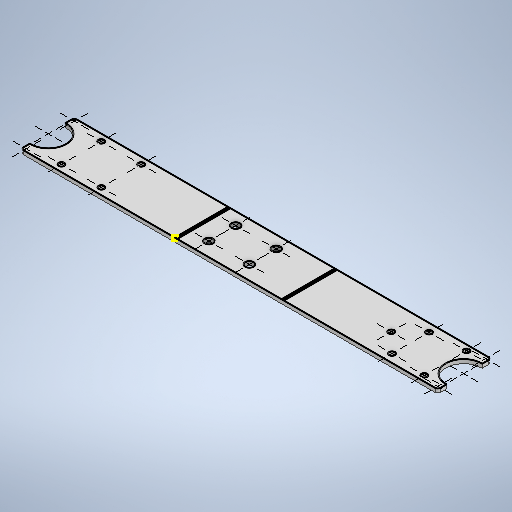
# Autodesk Inventor part: axis_21_top_frame
Saved by Autodesk Inventor 2026.1 (Build 301233000, 233)
## iProperties
Created: 2025-08-22
Part Number: axis_21_top_frame
Material: Generic
Document SubType Name: Modeling
Designer: LG
Density: 1 g/cm^3
Appearance: Default
Author: LG
Autodesk Inventor part; units mm, degrees
ref_plane "YZ Plane" through (0, 0, 0) normal (1, 0, 0) x (0, 1, 0)
ref_plane "XZ Plane" through (0, 0, 0) normal (0, 1, 0) x (-1, 0, 0)
ref_plane "XY Plane" through (0, 0, 0) normal (0, 0, 1) x (1, 0, 0)
sketch "Sketch1" plane through (0, 0, 0) normal (0, 1, 0) x (-1, 0, 0)
  line L0 (-40.8289, 0) -> (-40.8289, -20.14)
  line L1 (-0.4496, -20.14) -> (-0.4496, 0)
  circle A0 centre (45.43, -2.545) radius 1.05
  circle A1 centre (45.43, -17.595) radius 1.05
  circle A2 centre (30.33, -2.545) radius 1.05
  circle A3 centre (30.33, -17.595) radius 1.05
  circle A4 centre (-22.8893, -5.31) radius 1.55
  circle A5 centre (-22.8893, -15.45) radius 1.55
  circle A6 centre (-7.5893, -5.31) radius 1.55
  circle A7 centre (-7.5893, -15.45) radius 1.55
  circle A8 centre (-92.3086, -18.07) radius 1.05
  circle A9 centre (-92.3086, -2.07) radius 1.05
  circle A10 centre (-79.0886, -17.07) radius 1.05
  circle A11 centre (-79.0886, -3.07) radius 1.05
  circle A12 centre (-71.7886, -10.07) radius 1.05
  arc A13 (58.19, -3.325) -> (58.19, -16.815) centre (57.93, -10.07) ccw
  line L2 (58.19, -16.815) -> (58.19, -19.14)
  arc A14 (-99.4686, -16.815) -> (-99.4686, -3.325) centre (-99.2086, -10.07) ccw
  line L3 (-99.4686, -19.14) -> (-99.4686, -16.815)
  arc A15 (-99.4686, -19.14) -> (-98.4686, -20.14) centre (-98.4686, -19.14) ccw
  line L4 (57.19, -20.14) -> (-98.4686, -20.14)
  arc A16 (57.19, -20.14) -> (58.19, -19.14) centre (57.19, -19.14) ccw
  line L5 (58.19, -1) -> (58.19, -3.325)
  arc A17 (58.19, -1) -> (57.19, 0) centre (57.19, -1) ccw
  line L6 (-98.4686, 0) -> (57.19, 0)
  arc A18 (-98.4686, 0) -> (-99.4686, -1) centre (-98.4686, -1) ccw
  line L7 (-99.4686, -3.325) -> (-99.4686, -1)
  line L8 (-41.2786, -20.14) -> (-41.2786, 0)
  line L9 (-40.3793, 0) -> (-40.3793, -20.14)
  line L10 (-0.8993, -20.14) -> (-0.8993, 0)
  line L11 (0, 0) -> (0, -20.14)
  constraints: 24 end point, 19 centre point, 15 equal radius, 12 point on circle, 12 point on line, 12 tangent, 10 vertical, 7 parallel, 2 horizontal, 2 perpendicular, 63 other
extrude "Extrusion1" add sketch "Sketch1" against normal blind 1.5
body "Solid1"
